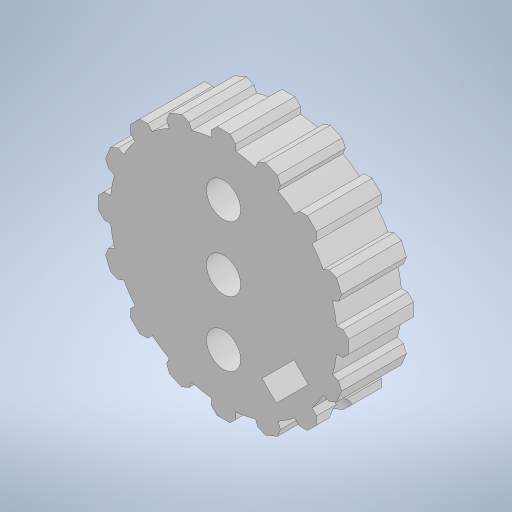
# Autodesk Inventor part: Деталь2
Saved by Autodesk Inventor 2023.1 (Build 271208000, 208)
## iProperties
Created: 2025-10-16
Part Number: Деталь2
Material: Типовые
Document SubType Name: Modeling
Designer: DELL
Density: 1 g/cm^3
Appearance: По умолчанию
Author: DELL
Autodesk Inventor part; units mm, degrees
ref_plane "YZ Plane" through (0, 0, 0) normal (1, 0, 0) x (0, 1, 0)
ref_plane "XZ Plane" through (0, 0, 0) normal (0, 1, 0) x (-1, 0, 0)
ref_plane "XY Plane" through (0, 0, 0) normal (0, 0, 1) x (1, 0, 0)
sketch "Эскиз1" plane through (0, 0, 0) normal (0, 0, 1) x (1, 0, 0)
  circle A0 centre (0, 0) radius 14
  line L0 (-1.5, 14.7194) -> (-1.5, 13.9194)
  line L1 (-1.5, 13.9194) -> (1.5, 13.9194)
  line L2 (1.5, 13.9194) -> (1.5, 14.7194)
  line L3 (0.8, 15.4194) -> (-0.8, 15.4194)
  line L4 (-1.5, 15.4194) -> (1.5, 13.9194) construction
  line L5 (-1.5, 13.9194) -> (1.5, 15.4194) construction
  line L6 (0, 0) -> (0, 20.7764) construction
  line L7 (-0.8, 15.4194) -> (-1.5, 14.7194)
  line L8 (0.8, 15.4194) -> (1.5, 14.7194)
  line L9 (-5.1616, 14.5518) -> (-6.6399, 13.9395)
  line L10 (-6.6399, 13.9395) -> (-7.0187, 13.0249)
  line L11 (-7.0187, 13.0249) -> (-6.7125, 12.2858)
  line L12 (-6.7125, 12.2858) -> (-3.9409, 13.4339)
  line L13 (-3.9409, 13.4339) -> (-4.2471, 14.173)
  line L14 (-5.1616, 14.5518) -> (-4.2471, 14.173)
  line L15 (-10.3375, 11.4689) -> (-11.4689, 10.3375)
  line L16 (-11.4689, 10.3375) -> (-11.4689, 9.3475)
  line L17 (-11.4689, 9.3475) -> (-10.9032, 8.7818)
  line L18 (-10.9032, 8.7818) -> (-8.7818, 10.9032)
  line L19 (-8.7818, 10.9032) -> (-9.3475, 11.4689)
  line L20 (-10.3375, 11.4689) -> (-9.3475, 11.4689)
  line L21 (-13.9395, 6.6399) -> (-14.5518, 5.1616)
  line L22 (-14.5518, 5.1616) -> (-14.173, 4.2471)
  line L23 (-14.173, 4.2471) -> (-13.4339, 3.9409)
  line L24 (-13.4339, 3.9409) -> (-12.2858, 6.7125)
  line L25 (-12.2858, 6.7125) -> (-13.0249, 7.0187)
  line L26 (-13.9395, 6.6399) -> (-13.0249, 7.0187)
  line L27 (-15.4194, 0.8) -> (-15.4194, -0.8)
  line L28 (-15.4194, -0.8) -> (-14.7194, -1.5)
  line L29 (-14.7194, -1.5) -> (-13.9194, -1.5)
  line L30 (-13.9194, -1.5) -> (-13.9194, 1.5)
  line L31 (-13.9194, 1.5) -> (-14.7194, 1.5)
  line L32 (-15.4194, 0.8) -> (-14.7194, 1.5)
  line L33 (-14.5518, -5.1616) -> (-13.9395, -6.6399)
  line L34 (-13.9395, -6.6399) -> (-13.0249, -7.0187)
  line L35 (-13.0249, -7.0187) -> (-12.2858, -6.7125)
  line L36 (-12.2858, -6.7125) -> (-13.4339, -3.9409)
  line L37 (-13.4339, -3.9409) -> (-14.173, -4.2471)
  line L38 (-14.5518, -5.1616) -> (-14.173, -4.2471)
  line L39 (-11.4689, -10.3375) -> (-10.3375, -11.4689)
  line L40 (-10.3375, -11.4689) -> (-9.3475, -11.4689)
  line L41 (-9.3475, -11.4689) -> (-8.7818, -10.9032)
  line L42 (-8.7818, -10.9032) -> (-10.9032, -8.7818)
  line L43 (-10.9032, -8.7818) -> (-11.4689, -9.3475)
  line L44 (-11.4689, -10.3375) -> (-11.4689, -9.3475)
  line L45 (-6.6399, -13.9395) -> (-5.1616, -14.5518)
  line L46 (-5.1616, -14.5518) -> (-4.2471, -14.173)
  line L47 (-4.2471, -14.173) -> (-3.9409, -13.4339)
  line L48 (-3.9409, -13.4339) -> (-6.7125, -12.2858)
  line L49 (-6.7125, -12.2858) -> (-7.0187, -13.0249)
  line L50 (-6.6399, -13.9395) -> (-7.0187, -13.0249)
  line L51 (-0.8, -15.4194) -> (0.8, -15.4194)
  line L52 (0.8, -15.4194) -> (1.5, -14.7194)
  line L53 (1.5, -14.7194) -> (1.5, -13.9194)
  line L54 (1.5, -13.9194) -> (-1.5, -13.9194)
  line L55 (-1.5, -13.9194) -> (-1.5, -14.7194)
  line L56 (-0.8, -15.4194) -> (-1.5, -14.7194)
  line L57 (5.1616, -14.5518) -> (6.6399, -13.9395)
  line L58 (6.6399, -13.9395) -> (7.0187, -13.0249)
  line L59 (7.0187, -13.0249) -> (6.7125, -12.2858)
  line L60 (6.7125, -12.2858) -> (3.9409, -13.4339)
  line L61 (3.9409, -13.4339) -> (4.2471, -14.173)
  line L62 (5.1616, -14.5518) -> (4.2471, -14.173)
  line L63 (10.3375, -11.4689) -> (11.4689, -10.3375)
  line L64 (11.4689, -10.3375) -> (11.4689, -9.3475)
  line L65 (11.4689, -9.3475) -> (10.9032, -8.7818)
  line L66 (10.9032, -8.7818) -> (8.7818, -10.9032)
  line L67 (8.7818, -10.9032) -> (9.3475, -11.4689)
  line L68 (10.3375, -11.4689) -> (9.3475, -11.4689)
  line L69 (13.9395, -6.6399) -> (14.5518, -5.1616)
  line L70 (14.5518, -5.1616) -> (14.173, -4.2471)
  line L71 (14.173, -4.2471) -> (13.4339, -3.9409)
  line L72 (13.4339, -3.9409) -> (12.2858, -6.7125)
  line L73 (12.2858, -6.7125) -> (13.0249, -7.0187)
  line L74 (13.9395, -6.6399) -> (13.0249, -7.0187)
  line L75 (15.4194, -0.8) -> (15.4194, 0.8)
  line L76 (15.4194, 0.8) -> (14.7194, 1.5)
  line L77 (14.7194, 1.5) -> (13.9194, 1.5)
  line L78 (13.9194, 1.5) -> (13.9194, -1.5)
  line L79 (13.9194, -1.5) -> (14.7194, -1.5)
  line L80 (15.4194, -0.8) -> (14.7194, -1.5)
  line L81 (14.5518, 5.1616) -> (13.9395, 6.6399)
  line L82 (13.9395, 6.6399) -> (13.0249, 7.0187)
  line L83 (13.0249, 7.0187) -> (12.2858, 6.7125)
  line L84 (12.2858, 6.7125) -> (13.4339, 3.9409)
  line L85 (13.4339, 3.9409) -> (14.173, 4.2471)
  line L86 (14.5518, 5.1616) -> (14.173, 4.2471)
  line L87 (11.4689, 10.3375) -> (10.3375, 11.4689)
  line L88 (10.3375, 11.4689) -> (9.3475, 11.4689)
  line L89 (9.3475, 11.4689) -> (8.7818, 10.9032)
  line L90 (8.7818, 10.9032) -> (10.9032, 8.7818)
  line L91 (10.9032, 8.7818) -> (11.4689, 9.3475)
  line L92 (11.4689, 10.3375) -> (11.4689, 9.3475)
  line L93 (6.6399, 13.9395) -> (5.1616, 14.5518)
  line L94 (5.1616, 14.5518) -> (4.2471, 14.173)
  line L95 (4.2471, 14.173) -> (3.9409, 13.4339)
  line L96 (3.9409, 13.4339) -> (6.7125, 12.2858)
  line L97 (6.7125, 12.2858) -> (7.0187, 13.0249)
  line L98 (6.6399, 13.9395) -> (7.0187, 13.0249)
  point P0 (0, 14.6694)
  point P1 (0, 14.6694)
  point P2 (-13.9194, 1.5)
  point P3 (-1.5, -13.9194)
  point P4 (13.9194, -1.5)
  dimension "d0" = 28
  dimension "d1" = 1.5
  dimension "d2" = 3
  dimension "d3" = 0.7
  dimension "d4" = 0.7
  dimension "d5" = 0.7
  dimension "d6" = 0.7
  dimension "d9" = 360
  constraints: 198 end point, 5 point on line, 3 midpoint, 2 parallel, 1 coincident, 1 perpendicular, 1 vertical, 197 other
  measures "d1" distance of L1.end L5.end
  measures "d2" distance of L5.end L4.start
  measures "d3" distance of L3.end L4.start
  measures "d4" distance of L0.start L4.start
  measures "d5" distance of L3.start L5.end
  measures "d6" distance of L2.end L5.end
extrude "Выдавливание1" add sketch "Эскиз1" along normal blind 8
sketch "Эскиз2" plane through (11.4689, -10.3375, 8) normal (0.7071, -0.7071, 0) x (-0.7071, -0.7071, 0)
  circle A0 centre (0.8, 3) radius 1.6
  line L0 (1.6, 0) -> (0, 0) projected
  point P0 (0.8, 8)
  point P1 (0.8, 0)
  dimension "d13" = 3.2
  dimension "d14" = 3
  constraints: 1 centre point, 1 midpoint
  measures "d13" diameter of A0
  measures "d14" distance of point (0.8, 0) A0.centre
extrude "Выдавливание2" cut sketch "Эскиз2" against normal blind 10
sketch "Эскиз3" plane through (0, 0, 8) normal (0, 0, 1) x (1, 0, 0)
  line L0 (11.4689, -10.3375) -> (10.3375, -11.4689) projected
  line L1 (10.9032, -10.9032) -> (0, 0) construction
  line L2 (6.5054, -10.4652) -> (10.4652, -6.5054)
  line L3 (10.4652, -6.5054) -> (8.6974, -4.7376)
  line L4 (8.6974, -4.7376) -> (4.7376, -8.6974)
  line L5 (4.7376, -8.6974) -> (6.5054, -10.4652)
  line L6 (6.5054, -10.4652) -> (8.6974, -4.7376) construction
  line L7 (10.4652, -6.5054) -> (4.7376, -8.6974) construction
  arc A0 (6.7125, -12.2858) -> (8.7818, -10.9032) centre (0, 0) ccw projected
  point P0 (7.6014, -7.6014)
  dimension "d17" = 5.6
  dimension "d18" = 2.5
  dimension "d19" = 12
  constraints: 14 end point, 3 midpoint, 3 perpendicular, 2 parallel, 1 point on line
  measures "d17" distance of L2.start L2.end
  measures "d18" distance of L3.end L2.end
  measures "d19" distance from line of A0.centre L2
extrude "Выдавливание3" cut sketch "Эскиз3" against normal blind 6
sketch "Эскиз4" plane through (0, 0, 8) normal (0, 0, 1) x (1, 0, 0)
  circle A0 centre (0, 0) radius 2.1
  circle A1 centre (0, 8) radius 2.1
  circle A2 centre (0, -8) radius 2.1
  dimension "d22" = 4.2
  dimension "d23" = 4.2
  dimension "d24" = 4.2
  dimension "d25" = 8
  dimension "d26" = 8
  constraints: 3 centre point, 1 coincident
  measures "d22" diameter of A0
  measures "d23" diameter of A1
  measures "d24" diameter of A2
  measures "d25" distance of point (0, 0) A1.centre
  measures "d26" distance of A2.centre point (0, 0)
extrude "Выдавливание4" cut sketch "Эскиз4" against normal blind 10
sketch "Эскиз5" plane through (0, 0, 0) normal (0, 0, -1) x (-1, 0, 0)
  circle A0 centre (0, 8) radius 2.1 projected
  line L0 (-2.0207, 4.5) -> (-4.0415, 8)
  line L1 (-4.0415, 8) -> (-2.0207, 11.5)
  line L2 (-2.0207, 11.5) -> (2.0207, 11.5)
  line L3 (2.0207, 11.5) -> (4.0415, 8)
  line L4 (4.0415, 8) -> (2.0207, 4.5)
  line L5 (2.0207, 4.5) -> (-2.0207, 4.5)
  circle A1 centre (0, -8) radius 2.1 projected
  line L6 (4.0415, -8) -> (2.0207, -11.5)
  line L7 (2.0207, -11.5) -> (-2.0207, -11.5)
  line L8 (-2.0207, -11.5) -> (-4.0415, -8)
  line L9 (-4.0415, -8) -> (-2.0207, -4.5)
  line L10 (-2.0207, -4.5) -> (2.0207, -4.5)
  line L11 (2.0207, -4.5) -> (4.0415, -8)
  point P0 (0, 0)
  point P1 (0, 11.5)
  point P2 (0, 4.5)
  dimension "d30" = 7
  dimension "d31" = 7
  constraints: 24 end point, 2 coincident, 2 midpoint, 26 other
  measures "d30" distance between parallel lines of L5 L2
  measures "d31" distance between parallel lines of L9 L6
extrude "Выдавливание5" cut sketch "Эскиз5" against normal blind 3.3
equation "\"d4\" = d3"
equation "\"d5\" = d3"
equation "\"d6\" = d5"
